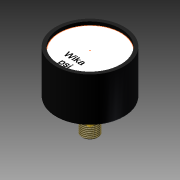
# Autodesk Inventor part: 9690242
Saved by Autodesk Inventor 2011 (Build 150239000, 239)
## iProperties
Category: Pneumatics
Company: Autodesk, Inc.
Shininess: 64.0
Length Units: 11269
Angle Units: 11279
Time Units: 11290
Mass Units: 11283
Length Display Precision: 3
Angle Display Precision: 2
Compacted: True
Part Number: 9690242
Document SubType Name: Modeling
Created: 2009-01-09
Manufacturer: Standard
Standards Organization: Custom
Catalog Web Link: www.wika.com
Description: Pressure Gauge
Vendor: WIKA
Density: 1 g/cm^3
Project: FIRST
Density: 0.0
Volumn: 0.0
Area: 0.0
PropertySet Name: Model Information
Control State: 0
Master: False
Checked Out: False
Title: Pressure Gauge
Author: Autodesk, Inc.
Autodesk Inventor part; units mm, degrees
ref_plane "YZ Plane" through (0, 0, 0) normal (1, 0, 0) x (0, 1, 0)
ref_plane "XZ Plane" through (0, 0, 0) normal (0, 1, 0) x (-1, 0, 0)
ref_plane "XY Plane" through (0, 0, 0) normal (0, 0, 1) x (1, 0, 0)
sketch "Sketch13" plane through (0, 0, 0) normal (0, 0, 1) x (1, 0, 0)
  circle A0 centre (0, 0) radius 20
  dimension "d46" = 40
  constraints: 1 centre point, 1 coincident
  measures "d46" diameter of A0
extrude "Extrusion13" add sketch "Sketch13" along normal blind 26
sketch "Sketch15" plane through (0, 0, 0) normal (0, 0, -1) x (-1, 0, 0)
  line L0 (-7, 7) -> (7, 7)
  line L1 (7, 7) -> (7, -7)
  line L2 (7, -7) -> (-7, -7)
  line L3 (-7, -7) -> (-7, 7)
  line L4 (-28, 0) -> (28, 0) projected
  line L5 (0, -28) -> (0, 28) projected
  dimension "d52" = 14
  dimension "d53" = 14
  constraints: 8 end point, 2 parallel, 1 horizontal, 1 perpendicular, 2 other
  measures "d52" distance of L2.end L0.start
  measures "d53" distance of L0.start L0.end
extrude "Extrusion15" add sketch "Sketch15" along normal blind 8
sketch "Sketch16" plane through (0, 0, -8) normal (0, 0, -1) x (-1, 0, 0)
  circle A0 centre (0, 0) radius 4.7625
  dimension "d58" = 9.525
  constraints: 1 centre point, 1 coincident
  measures "d58" diameter of A0
extrude "Extrusion16" add sketch "Sketch16" along normal blind 10
thread "Thread3" size "1/8" designation "1/8 - 27 NPT" standard "NPT" full length
sketch "Sketch18" plane through (0, 0, 26) normal (0, 0, 1) x (1, 0, 0)
  circle A0 centre (0, 0) radius 20 projected
  circle A1 centre (0, 0) radius 18
  dimension "d66" = 2
  constraints: 1 centre point
  measures "d66" radial gap between concentric circles of A0 A1
extrude "Extrusion18" cut sketch "Sketch18" against normal blind 2 contours A1
sketch "Sketch20" plane through (0, 0, -18) normal (0, 0, -1) x (-1, 0, 0)
  circle A0 centre (0, 0) radius 4.7625 projected
  circle A1 centre (0, 0) radius 1.5
  dimension "d75" = 3
  constraints: 1 centre point, 1 coincident
  measures "d75" diameter of A1
extrude "Extrusion19" cut sketch "Sketch20" against normal blind 10 contours A1
sketch "Sketch19" plane through (0, 0, 24) normal (0, 0, 1) x (1, 0, 0)
  circle A0 centre (0, 0) radius 18 projected
  line L0 (-6.3869, -6.5985) -> (5.7442, -6.5985) construction
  line L1 (5.7442, -6.5985) -> (5.7442, -16.6783) construction
  line L2 (5.7442, -16.6783) -> (-6.3869, -16.6783) construction
  line L3 (-6.3869, -16.6783) -> (-6.3869, -6.5985) construction
  constraints: 2 other
chamfer "Chamfer1" distance 0.5 angle 45 1 edges at (4.7625, 0, -18)
fillet "Fillet5" radius 1 1 edges at (-20, 0, 0)
body "Solid1"
